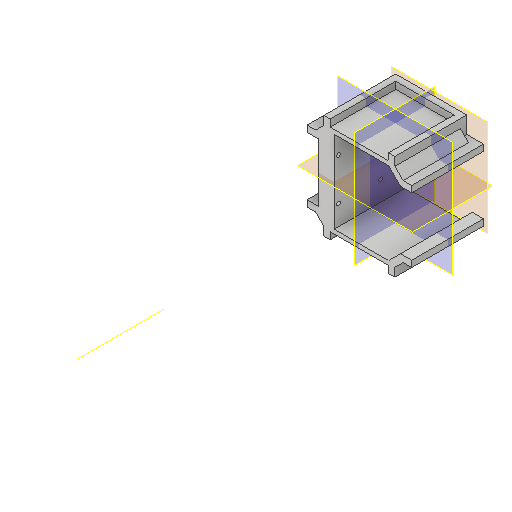
# Autodesk Inventor part: 30_Cube_SQUID_Z_Focus_base_v3
Saved by Autodesk Inventor 2022 (Build 260153000, 153)
## iProperties
Created: 2021-04-25
Part Number: 30_Cube_SQUID_Z_Focus_base_v3
Material: Generic
Document SubType Name: Modeling
Designer: diederichbenedict
Density: 1 g/cm^3
Appearance: Smooth - White
Author: diederichbenedict
Autodesk Inventor part; units mm, degrees
ref_plane "YZ Plane" through (0, 0, 0) normal (1, 0, 0) x (0, 1, 0)
ref_plane "XZ Plane" through (0, 0, 0) normal (0, 1, 0) x (-1, 0, 0)
ref_plane "Work Plane1" through (0, 0, -1) normal (0, 0, 1) x (1, 0, 0)
sketch "Sketch1" plane through (0, 0, -1) normal (0, 0, 1) x (1, 0, 0)
  line L0 (24.85, 16.87) -> (16.87, 16.87)
  line L1 (16.87, 16.87) -> (16.87, -16.87)
  line L2 (16.87, -16.87) -> (24.85, -16.87)
  line L3 (24.85, -16.87) -> (24.85, 16.87)
  line L4 (-16.87, 24.85) -> (16.87, 24.85)
  line L5 (16.87, 24.85) -> (16.87, 13.87)
  line L6 (16.87, 13.87) -> (-16.87, 13.87)
  line L7 (-16.87, 13.87) -> (-16.87, 24.85)
  line L8 (-16.87, 16.87) -> (-24.85, 16.87)
  line L9 (-24.85, 16.87) -> (-24.85, -16.87)
  line L10 (-24.85, -16.87) -> (-16.87, -16.87)
  line L11 (-16.87, -16.87) -> (-16.87, 16.87)
  line L12 (-16.87, -24.85) -> (16.87, -24.85)
  line L13 (16.87, -24.85) -> (16.87, -13.87)
  line L14 (16.87, -13.87) -> (-16.87, -13.87)
  line L15 (-16.87, -13.87) -> (-16.87, -24.85)
  line L16 (-16.87, 13.87) -> (3.07, 13.87)
  line L17 (3.07, -13.87) -> (-16.87, -13.87)
  line L18 (-16.87, -13.87) -> (-16.87, 13.87)
  line L19 (-16.87, 7.9971) -> (-16.87, -7.9971)
  circle A0 centre (-0.83, -7.7) radius 1 projected
  circle A1 centre (14.57, -7.7) radius 1 projected
  circle A2 centre (14.57, 7.7) radius 1 projected
  circle A3 centre (-0.83, 7.7) radius 1 projected
  circle A4 centre (6.87, 0) radius 8 construction
  circle A5 centre (6.87, 0) radius 9.25
  dimension "d6" = 3
  dimension "d7" = 3
  dimension "d123" = 18.5
  constraints: 40 end point, 9 parallel, 7 point on line, 5 horizontal, 4 perpendicular, 1 centre point, 1 coincident, 1 collinear
  measures "d6" distance between parallel lines of L8 L6
  measures "d7" distance between parallel lines of L10 L14
  measures "d123" diameter of A5
extrude "Extrusion1" add sketch "Sketch1" along normal blind 3
chamfer "Chamfer1" distance 3.9 angle 45 3 edges at (16.87, -16.87, 0.5) (-16.87, -16.87, 0.5) (-16.87, 16.87, 0.5)
sketch "Sketch2" plane through (0, 0, 2) normal (0, 0, 1) x (1, 0, 0)
  line L0 (16.87, 16.87) -> (16.87, 24.85) projected
  line L1 (-16.87, -20.77) -> (-16.87, -24.85) projected
  line L2 (-16.87, -24.85) -> (16.87, -24.85) projected
  line L3 (16.87, -24.85) -> (16.87, -20.77) projected
  line L4 (20.77, -16.87) -> (16.87, -20.77) projected
  line L5 (20.77, -16.87) -> (24.85, -16.87) projected
  line L6 (24.85, -16.87) -> (24.85, 16.87) projected
  line L7 (24.85, 16.87) -> (16.87, 16.87) projected
  line L8 (16.87, 24.85) -> (-16.87, 24.85) projected
  line L9 (-16.87, 24.85) -> (-16.87, 20.77) projected
  line L10 (-20.77, 16.87) -> (-16.87, 20.77) projected
  line L11 (-20.77, 16.87) -> (-24.85, 16.87) projected
  line L12 (-24.85, 16.87) -> (-24.85, -16.87) projected
  line L13 (-24.85, -16.87) -> (-20.77, -16.87) projected
  line L14 (-16.87, -20.77) -> (-20.77, -16.87) projected
  line L15 (13.8689, -19.5269) -> (13.8689, -21.8489)
  line L16 (-13.8689, -21.8489) -> (-13.8689, -19.5269)
  line L17 (-13.8689, -19.5269) -> (-19.5269, -13.8689)
  line L18 (-19.5269, -13.8689) -> (-21.8489, -13.8689)
  line L19 (-21.8489, 13.8689) -> (-19.5269, 13.8689)
  line L20 (-19.5269, 13.8689) -> (-13.8689, 19.5269)
  line L21 (-13.8689, 19.5269) -> (-13.8689, 21.8489)
  line L22 (13.8689, 21.8489) -> (13.8689, 19.5269)
  line L23 (13.8689, 19.5269) -> (19.5269, 13.8689)
  line L24 (19.5269, 13.8689) -> (21.8489, 13.8689)
  line L25 (21.8489, -13.8689) -> (19.5269, -13.8689)
  line L26 (19.5269, -13.8689) -> (13.8689, -19.5269)
  line L27 (13.8689, -21.8489) -> (13.8689, -24.85)
  line L28 (16.87, -24.85) -> (-16.87, -24.85) projected
  line L29 (21.8489, -13.8689) -> (24.85, -13.8689)
  line L30 (24.85, -16.87) -> (24.85, 16.87) projected
  line L31 (21.8489, 13.8689) -> (24.85, 13.8689)
  line L32 (13.8689, 21.8489) -> (13.8689, 24.85)
  line L33 (-13.8689, 21.8489) -> (-13.8689, 24.85)
  line L34 (-21.8489, 13.8689) -> (-24.85, 13.8689)
  line L35 (-21.8489, -13.8689) -> (-24.85, -13.8689)
  line L36 (-13.8689, -21.8489) -> (-13.8689, -24.85)
  line L37 (13.8689, -21.8489) -> (11.5469, -21.8489)
  line L38 (-11.5469, -21.8489) -> (-13.8689, -21.8489)
  line L39 (21.8489, 13.8689) -> (21.8489, 11.5469)
  line L40 (21.8489, -11.5469) -> (21.8489, -13.8689)
  line L41 (-21.8489, -13.8689) -> (-21.8489, -11.5469)
  line L42 (-21.8489, 11.5469) -> (-21.8489, 13.8689)
  line L43 (-13.8689, 21.8489) -> (-11.5469, 21.8489)
  line L44 (11.5469, 21.8489) -> (13.8689, 21.8489)
  point P0 (0, 0)
  dimension "d13" = 3.0011
  constraints: 56 end point, 20 point on line, 3 perpendicular, 1 parallel, 5 other
  measures "d13" distance between parallel lines of L3 L15
ref_plane "Work Plane2" through (-16.97, -24.85, 34.1) normal (0, 0, -1) x (0, 1, 0)
extrude "Extrusion2" add sketch "Sketch2" along normal blind 31.1 contours L6 L5 L4 L3 L2 L27 L15 L26 L25 L29
pattern_circular "Circular Pattern1" count 4 over 360 about axis through (0, 0, 146.63) along (0, 0, -1) of "Extrusion2"
ref_plane "Work Plane9" through (-16.87, 0, -1) normal (0, 1, 0) x (1, 0, 0)
ref_plane "Work Plane10" through (0, -16.87, -1) normal (-1, 0, 0) x (0, 0, 1)
ref_plane "Work Plane11" through (0, 0, 16.05) normal (0, 0, -1) x (-1, 0, 0)
sketch "Sketch23" plane through (0, 0, 2) normal (0, 0, 1) x (1, 0, 0)
  line L0 (13.8689, 19.5269) -> (13.8689, 24.85) projected
  line L1 (13.8689, 24.85) -> (-13.8689, 24.85) projected
  line L2 (-13.8689, 24.85) -> (-13.8689, 19.5269) projected
  line L3 (-13.8689, 19.5269) -> (-19.5269, 13.8689) projected
  line L4 (-19.5269, 13.8689) -> (-24.85, 13.8689) projected
  line L5 (-24.85, 13.8689) -> (-24.85, -13.8689) projected
  line L6 (-24.85, -13.8689) -> (-19.5269, -13.8689) projected
  line L7 (-19.5269, -13.8689) -> (-13.8689, -19.5269) projected
  line L8 (-13.8689, -19.5269) -> (-13.8689, -24.85) projected
  line L9 (-13.8689, -24.85) -> (13.8689, -24.85) projected
  line L10 (13.8689, -24.85) -> (13.8689, -19.5269) projected
  line L11 (13.8689, -19.5269) -> (19.5269, -13.8689) projected
  line L12 (19.5269, -13.8689) -> (24.85, -13.8689) projected
  line L13 (24.85, -13.8689) -> (24.85, 13.8689) projected
  line L14 (24.85, 13.8689) -> (19.5269, 13.8689) projected
  line L15 (19.5269, 13.8689) -> (13.8689, 19.5269) projected
  circle A0 centre (-0.83, 7.7) radius 1 projected
  circle A1 centre (14.57, 7.7) radius 1 projected
  circle A2 centre (14.57, -7.7) radius 1 projected
  circle A3 centre (-0.83, -7.7) radius 1 projected
  line L16 (-12, 7.4) -> (-12, 12) projected
  line L17 (-12, -12) -> (-12, -7.4) projected
  line L18 (-13.8689, -19.5269) -> (-19.5269, -13.8689) projected
  line L19 (-12, 19.5269) -> (-13.8689, 19.5269)
  line L20 (-13.8689, 19.5269) -> (-13.8689, -19.5269)
  line L21 (-13.8689, -19.5269) -> (-12, -19.5269)
  line L22 (-12, -19.5269) -> (-12, 19.5269)
  line L23 (-19.5269, 13.8689) -> (-19.5269, -13.8689)
  line L24 (19.5269, 13.8689) -> (13.8689, 19.5269) projected
  line L25 (-13.8689, 24.85) -> (-13.8689, 19.5269) projected
  line L26 (13.8689, 19.5269) -> (-13.8689, 19.5269)
  line L27 (-13.8689, 19.5269) -> (-13.8689, 21.5269)
  line L28 (-13.8689, 21.5269) -> (13.8689, 21.5269)
  line L29 (13.8689, 21.5269) -> (13.8689, 19.5269)
  line L30 (13.8689, -19.5269) -> (13.8689, -24.85) projected
  line L31 (-13.8689, -19.5269) -> (13.8689, -19.5269)
  line L32 (13.8689, -19.5269) -> (13.8689, -21.5269)
  line L33 (13.8689, -21.5269) -> (-13.8689, -21.5269)
  line L34 (-13.8689, -21.5269) -> (-13.8689, -19.5269)
  point P0 (0, 0)
  point P1 (-12, -7.4)
  point P2 (-12, 12)
  point P3 (13.8689, -21.5269)
  point P4 (13.8689, 21.5269)
  point P5 (-13.8689, 21.5269)
  dimension "d114" = 2
  dimension "d115" = 2
  constraints: 26 end point, 6 parallel, 3 horizontal, 3 perpendicular, 2 point on line, 1 vertical
  measures "d114" distance of L26.end L27.end
  measures "d115" distance of L31.end L32.end
extrude "Extrusion19" add sketch "Sketch23" along normal up to surface (31.1 mm away) contours L26 L19 L2 L28 L0 | L22 L16 L17 L21 L20 L19 | L20 L7 L23 L3 | L21 L31 L10 L33 L8
hole "Hole4" at (-19.5269, 10, 31.05) at (-19.5269, -10, 31.05) at (-19.5269, 10, 11.05) at (-19.5269, -10, 11.05) direction (1, 0, 0) diameter 1.8 depth 15 tip angle 118
sketch "Sketch25" plane through (0, 0, 2) normal (0, 0, 1) x (1, 0, 0)
  circle A0 centre (-0.83, -7.7) radius 1 projected
  circle A1 centre (14.57, -7.7) radius 1 projected
  circle A2 centre (14.57, 7.7) radius 1 projected
  circle A3 centre (-0.83, 7.7) radius 1 projected
  circle A4 centre (6.87, 0) radius 9.25 projected
  line L0 (13.8689, 19.5269) -> (-12, 19.5269) projected
  line L1 (-12, 19.5269) -> (-12, -19.5269) projected
  line L2 (-12, -19.5269) -> (13.8689, -19.5269) projected
  line L3 (13.8689, -19.5269) -> (19.5269, -13.8689) projected
  line L4 (19.5269, -13.8689) -> (24.85, -13.8689) projected
  line L5 (24.85, -13.8689) -> (24.85, 13.8689) projected
  line L6 (24.85, 13.8689) -> (19.5269, 13.8689) projected
  line L7 (19.5269, 13.8689) -> (13.8689, 19.5269) projected
  point P0 (0, 0)
extrude "Extrusion20" cut sketch "Sketch25" against normal through all
body "Solid1"
